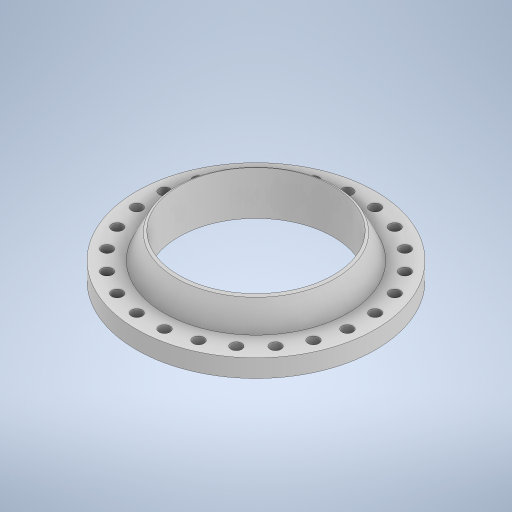
# Autodesk Inventor part: ANSI-B300-24W
Saved by Autodesk Inventor 2023 (Build 270158000, 158)
## iProperties
Created: 2023-11-03
Part Number: ANSI-B300-24W
Material: Generic
Document SubType Name: Modeling
Designer: Admin
Density: 1 g/cm^3
Appearance: Default
Author: Admin
Autodesk Inventor part; units mm, degrees
ref_plane "YZ Plane" through (0, 0, 0) normal (1, 0, 0) x (0, 1, 0)
ref_plane "XZ Plane" through (0, 0, 0) normal (0, 1, 0) x (-1, 0, 0)
ref_plane "XY Plane" through (0, 0, 0) normal (0, 0, 1) x (1, 0, 0)
sketch "Sketch1" plane through (0, 0, 0) normal (0, 0, 1) x (1, 0, 0)
  line L0 (0, 0) -> (0, 168.2115) construction
  line L1 (-295.275, 168.2115) -> (-295.275, 0)
  line L2 (-295.275, 0) -> (-350.774, 0)
  line L3 (-350.774, 0) -> (-350.774, 1.5875)
  line L4 (-350.774, 1.5875) -> (-457.2, 1.5875)
  line L5 (-457.2, 1.5875) -> (-457.2, 69.9135)
  line L6 (-457.2, 69.9135) -> (-350.774, 69.9135)
  line L7 (-350.774, 69.9135) -> (-304.8, 162.7122)
  line L8 (-304.8, 162.7122) -> (-295.275, 168.2115)
  line L9 (-406.4, 69.9135) -> (-406.4, 1.5875) construction
  dimension "WB" = 590.55
  dimension "d1" = 1.5875
  dimension "WL" = 166.624
  dimension "Thickness" = 68.326
  dimension "R" = 701.548
  dimension "OD" = 914.4
  dimension "HB" = 701.548
  dimension "HT" = 609.6
  dimension "d8" = 60
  dimension "BC" = 812.8
  constraints: 20 end point, 5 vertical, 3 horizontal, 2 horizontal alignment, 2 point on line
  measures "WB" diameter of L1 L0
  measures "d1" distance between parallel lines of L2 L4
  measures "WL" distance from line of L1.start L4
  measures "Thickness" distance of L4.end L5.end
  measures "R" diameter of L3 L0
  measures "OD" diameter of L5 L0
  measures "HB" diameter of L6.end L0
  measures "HT" diameter of L7.end L0
  measures "d8" angle of L8 L1
  measures "BC" diameter of L9 L0
revolve "Revolution1" add sketch "Sketch1" angle 360 about axis through (0, 0, 0) along (0, 1, 0)
sketch "Sketch2" plane through (0, 69.9135, 0) normal (0, 1, 0) x (1, 0, 0)
  line L0 (0, 0) -> (0, 457.2) construction
  circle A0 centre (0, 0) radius 457.2 projected
  line L1 (0, 0) -> (53.0458, 402.9232) construction
  dimension "d11" = 7.5
  dimension "d12" = 406.4
  constraints: 4 end point, 1 coincident, 1 vertical, 1 vertical alignment, 1 other
  measures "d11" angle of L1 L0
  measures "d12" distance of L1.start L1.end
hole "Hole1" at (53.0458, 69.9135, -402.9232) direction (0, -1, 0) diameter 41.402 depth 68.326
pattern_circular "Circular Pattern1" count 24 over 360 about axis through (0, -10, 0) along (0, 1, 0) of "Hole1"
equation "\"d12\" = 0.5 * BC"
body "Solid1"
